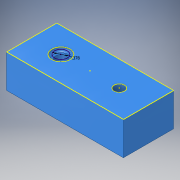
# Autodesk Inventor part: AirPressureAndValve
Saved by Autodesk Inventor 2018 (Build 220112000, 112)
## iProperties
Created: 2020-03-27
Part Number: AirPressureAndValve
Material: Generic
Document SubType Name: Modeling
Designer: emile
Density: 1 g/cm^3
Appearance: Cyan
Author: emile
Autodesk Inventor part; units mm, degrees
ref_plane "YZ Plane" through (0, 0, 0) normal (1, 0, 0) x (0, 1, 0)
ref_plane "XZ Plane" through (0, 0, 0) normal (0, 1, 0) x (-1, 0, 0)
ref_plane "XY Plane" through (0, 0, 0) normal (0, 0, 1) x (1, 0, 0)
sketch "Sketch1" plane through (0, 0, 0) normal (0, 1, 0) x (-1, 0, 0)
  line L0 (-44.45, -19.05) -> (44.45, -19.05)
  line L1 (44.45, -19.05) -> (44.45, 19.05)
  line L2 (44.45, 19.05) -> (-44.45, 19.05)
  line L3 (-44.45, 19.05) -> (-44.45, -19.05)
  line L4 (-44.45, -19.05) -> (44.45, 19.05) construction
  line L5 (44.45, -19.05) -> (-44.45, 19.05) construction
  circle A0 centre (22.225, 0) radius 3.9688
  circle A1 centre (-22.225, 0) radius 3.9688
  circle A2 centre (22.225, 0) radius 12.7
  circle A3 centre (-22.225, 0) radius 12.7
  point P0 (0, 0)
  point P1 (0, 0)
  point P2 (0, 0)
  dimension "d3" = 38.1
  dimension "d4" = 88.9
  dimension "d20" = 7.9375
  dimension "d21" = 25.4
  dimension "d22" = 22.225
  dimension "d23" = 22.225
  constraints: 12 end point, 4 centre point, 4 midpoint, 2 coincident, 2 equal radius, 2 horizontal alignment, 2 parallel, 1 horizontal, 1 perpendicular
  measures "d3" distance of L0.end L1.end
  measures "d4" distance of L0.start L0.end
  measures "d20" diameter of A0
  measures "d21" diameter of A2
  measures "d22" distance of point (0, 0) A2.centre
  measures "d23" distance of point (0, 0) A3.centre
extrude "Extrusion5" add sketch "Sketch1" along normal blind 25.4 contours L3 L2 L1 L0 | A2 | A3
sketch "Sketch8" plane through (0, 0, 0) normal (0, 0, 1) x (1, 0, 0)
  line L0 (44.45, 25.4) -> (-44.45, 25.4) projected
  circle A0 centre (-27.9591, 24.13) radius 1.7653
  line L1 (-26.1938, 25.4) -> (-18.2563, 25.4) projected
  line L2 (-18.2563, 0) -> (-26.1938, 0) projected
  line L3 (-26.1938, 0) -> (-26.1938, 25.4) projected
  line L4 (-18.2563, 0) -> (-18.2563, 25.4) projected
  line L5 (-22.225, 25.4) -> (-22.225, 0) construction
  line L6 (-44.45, 25.4) -> (-44.45, 27.8765) construction
  line L7 (-27.9591, 22.3647) -> (-22.225, 22.3647)
  line L8 (-26.7329, 25.4) -> (-22.225, 25.4) construction
  line L9 (-22.225, 22.3647) -> (-22.225, 25.4)
  line L10 (-22.225, 25.4) -> (-26.7329, 25.4)
  point P0 (0, 0)
  dimension "d34" = 3.5306
  dimension "d35" = 1.27
  constraints: 12 end point, 3 collinear, 2 midpoint, 2 point on circle, 2 point on line, 2 tangent, 1 centre point, 1 perpendicular, 1 vertical
  measures "d34" diameter of A0
  measures "d35" distance from line of L0 A0.centre
revolve "Revolution1" cut sketch "Sketch8" angle 360 about axis through (-22.225, 25.4, 0) along (0, -1, 0) contours L9 L7 L3 L0 | L3 A0 L0 | A0 L0 | L0 A0 | L3 L7 A0
sketch "Sketch9" plane through (0, 25.4, 0) normal (0, 1, 0) x (1, 0, 0)
  circle A0 centre (-22.225, 0) radius 6.9602 projected
  circle A1 centre (22.225, 0) radius 3.9687 projected
  line L0 (44.45, 19.05) -> (-44.45, 19.05) projected
  line L1 (-44.45, 19.05) -> (-44.45, -19.05) projected
  line L2 (-44.45, -19.05) -> (44.45, -19.05) projected
  line L3 (44.45, -19.05) -> (44.45, 19.05) projected
  circle A2 centre (-22.225, 0) radius 4.8006
  point P0 (0, 0)
  dimension "d37" = 9.6012
  constraints: 1 centre point, 1 coincident
  measures "d37" diameter of A2
equation "\"d23\" = d22"
body "Solid2"
